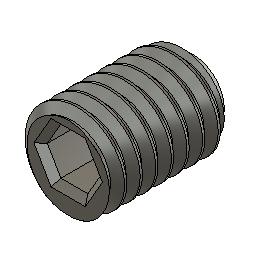
Poke_v15 (Autodesk Fusion 360 archive; units mm, degrees)
design "Set Screw m3x4"
Autodesk Fusion 360 part; units mm, degrees
sketch "Sketch1" plane through (0, 0, 0) normal (0, 0, 1) x (1, 0, 0)
  circle A0 centre (0, 0) radius 1.5
  line L0 (-0.433, 0.75) -> (-0.866, 0)
  line L1 (-0.866, 0) -> (-0.433, -0.75)
  line L2 (-0.433, -0.75) -> (0.433, -0.75)
  line L3 (0.433, -0.75) -> (0.866, 0)
  line L4 (0.866, 0) -> (0.433, 0.75)
  line L5 (0.433, 0.75) -> (-0.433, 0.75)
  dimension "d1" = 1.5
  dimension "d2" = 3
  constraint coincident A0.centre origin
  measures "d1" distance of L2 L5
  measures "d2" diameter of A0
extrude "Extrude1" add sketch "Sketch1" against normal blind 4 contours A0 | L0 L1 L2 L3 L4 L5
sketch "Sketch2" plane through (0, 0, 0) normal (0, 1, 0) x (1, 0, 0)
  line L0 (1.5, 4) -> (-1.5, 4)
  line L1 (-1.5, 0) -> (1.5, 0)
  line L2 (1, 4) -> (1.5, 3.5)
  line L3 (1.5, 3.5) -> (1.5, 4)
  dimension "d6" = 45
  dimension "d7" = 0.5
  constraint coincident L0 L2.start
  constraint coincident L0.start L3.end
  constraint vertical L3
  measures "d6" angle of L0 L2
  measures "d7" distance of L2.end L0.start
thread "Thread1" "ISO Metric profile 3.0 M3x0.5 6g" major diameter 2.927 minor diameter 2.3555 pitch 0.5 angle 60 modelled right hand crest width 0.0713 on face at (1.4981, -0.0748, -2.6667) crest through (1.4635, 0, 0.125)
extrude "Extrude2" cut sketch "Sketch2" along normal blind 0.039
revolve "Revolve1" cut sketch "Sketch2" angle 360 about axis through (0, 0, 1.75) along (0, 0, 1)
extrude "Extrude3" cut sketch "Sketch1" against normal blind 3 contours L0 L1 L2 L3 L4 L5
chamfer "Chamfer2" distance 0.2 angle 45 6 edges at (0, 0.75, 0) (0.6495, 0.375, 0) (0.6495, -0.375, 0) (0, -0.75, 0) (-0.6495, -0.375, 0) (-0.6495, 0.375, 0)
